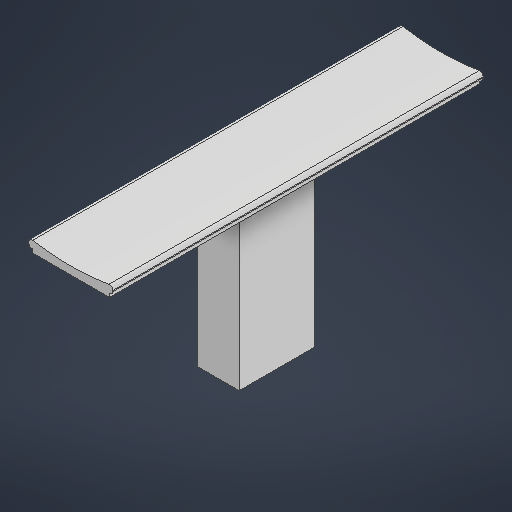
# Autodesk Inventor part: Patient_table
Saved by Autodesk Inventor 2026 (Build 300175000, 175)
## iProperties
Created: 2025-04-14
Part Number: Patient_table
Material: Generic
Document SubType Name: Modeling
Designer: aksha
Density: 1 g/cm^3
Appearance: Default
Author: aksha
Autodesk Inventor part; units mm, degrees
ref_plane "YZ Plane" through (0, 0, 0) normal (1, 0, 0) x (0, 1, 0)
ref_plane "XZ Plane" through (0, 0, 0) normal (0, 1, 0) x (-1, 0, 0)
ref_plane "XY Plane" through (0, 0, 0) normal (0, 0, 1) x (1, 0, 0)
sketch "Sketch1" plane through (0, 0, 0) normal (0, 0, 1) x (1, 0, 0)
  line L0 (-250, -15) -> (250, -15)
  line L1 (250, -15) -> (250, 35)
  line L2 (-250, 35) -> (-250, -15)
  line L3 (-250, -15) -> (250, 35) construction
  line L4 (250, -15) -> (-250, 35) construction
  arc A0 (-250, 35) -> (250, 35) centre (0, 1314.7822) ccw
  point P0 (0, 10)
  dimension "d6" = 500
  dimension "d7" = 50
  constraints: 10 end point, 2 midpoint, 2 point on circle, 1 centre point, 1 horizontal, 1 parallel, 1 perpendicular
  measures "d6" distance of L1.end L2.start
  measures "d7" distance of L1.end L0.end
extrude "Extrusion1" add sketch "Sketch1" along normal blind 2200
fillet "Fillet1" radius 20 1 edges at (250, 35, 1100)
fillet "Fillet2" radius 20 1 edges at (250, -15, 1100)
fillet "Fillet3" radius 20 2 edges at (-250, 35, 1100) (-250, -15, 1100)
sketch "Sketch2" plane through (230, -15, 0) normal (0, -1, 0) x (1, 0, 0)
  line L0 (0, 2200) -> (0, 0) projected
  line L1 (-456.5256, 0) -> (-3.4744, 0) projected
  line L2 (0, 2200) -> (-456.5256, 2200)
  line L3 (-456.5256, 2200) -> (-456.5256, 0)
  line L4 (-456.5256, 0) -> (0, 0)
  line L5 (0, 0) -> (0, 2200)
  line L6 (-103.2628, 1325) -> (-353.2628, 1325)
  line L7 (-353.2628, 1325) -> (-353.2628, 875)
  line L8 (-353.2628, 875) -> (-103.2628, 875)
  line L9 (-103.2628, 875) -> (-103.2628, 1325)
  line L10 (-103.2628, 1325) -> (-353.2628, 875) construction
  line L11 (-353.2628, 1325) -> (-103.2628, 875) construction
  point P0 (-230, 0)
  point P1 (-228.2628, 1100)
  dimension "d15" = 250
  dimension "d16" = 450
  constraints: 20 end point, 4 parallel, 2 horizontal, 2 midpoint, 2 perpendicular
  measures "d15" distance of L8.end L7.end
  measures "d16" distance of L7.end L6.end
extrude "Extrusion2" add sketch "Sketch2" along normal blind 20 contours L0 L4 L1 L3 L2 | L9 L8 L7 L6
sketch "Sketch3" plane through (230, -35, 0) normal (0, -1, 0) x (1, 0, 0)
  point P0 (-230, 0)
sketch "Sketch4" plane through (230, -35, 0) normal (0, -1, 0) x (1, 0, 0)
  line L0 (-105, 1325) -> (-355, 1325)
  line L1 (-355, 1325) -> (-355, 875)
  line L2 (-355, 875) -> (-105, 875)
  line L3 (-105, 875) -> (-105, 1325)
  line L4 (-105, 1325) -> (-355, 875) construction
  line L5 (-355, 1325) -> (-105, 875) construction
  point P0 (-230, 0)
  point P1 (-230, 1100)
  dimension "d17" = 250
  dimension "d18" = 450
  constraints: 12 end point, 2 midpoint, 2 parallel, 1 horizontal, 1 perpendicular
  measures "d17" distance of L2.end L1.end
  measures "d18" distance of L1.end L0.end
extrude "Extrusion3" add sketch "Sketch4" along normal blind 970
body "Solid1"
